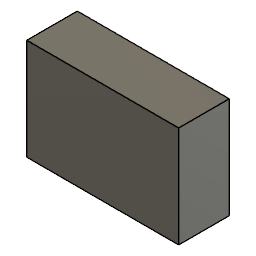
replay (Autodesk Fusion 360 design; units mm, degrees)
Autodesk Fusion 360 part; units mm, degrees
sketch "草图1" plane through (0, 0, 0) normal (0, 0, 1) x (1, 0, 0)
  line L0 (60, 0) -> (60, 40)
  line L1 (60, 40) -> (0, 40)
  line L2 (0, 40) -> (0, 0)
  line L3 (0, 0) -> (60, 0)
extrude "拉伸1" add sketch "草图1" along normal blind 20
